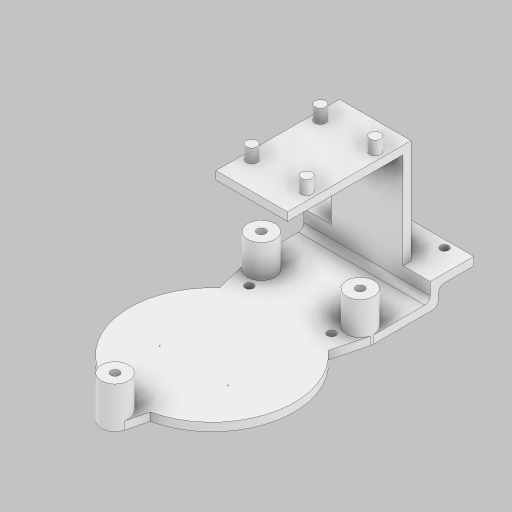
# Autodesk Inventor part: BASE_LIDAR_V4
Saved by Autodesk Inventor 2024.2 (Build 282272000, 272)
## iProperties
Created: 2024-07-17
Part Number: BASE_LIDAR_V4
Material: ABS Plastic
Document SubType Name: Modeling
Designer: jrcer
Density: 1.06 g/cm^3
Appearance: Smooth - White
Mass: 26.2686 g
Surface Area: 178.873 cm^2
Volume: 24.7817 cm^3
Author: jrcer
Autodesk Inventor part; units mm, degrees
ref_plane "YZ Plane" through (0, 0, 0) normal (1, 0, 0) x (0, 1, 0)
ref_plane "XZ Plane" through (0, 0, 0) normal (0, 1, 0) x (-1, 0, 0)
ref_plane "XY Plane" through (0, 0, 0) normal (0, 0, 1) x (1, 0, 0)
sketch "Sketch1" plane through (0, 0, 0) normal (0, 1, 0) x (-1, 0, 0)
  circle A0 centre (0, 35.3) radius 1.55
  circle A1 centre (18, -36) radius 1.55
  circle A2 centre (-18, -36) radius 1.55
  circle A3 centre (0, 35.3) radius 5
  circle A4 centre (18, -36) radius 5
  circle A5 centre (-18, -36) radius 5
  point P0 (0, 0)
  dimension "d0" = 35.3
  dimension "d1" = 36
  dimension "d2" = 3.1
  dimension "d3" = 10
  dimension "d4" = 36
  dimension "d5" = 18
  constraints: 6 centre point, 4 equal radius, 3 coincident, 1 horizontal alignment, 1 vertical alignment
  measures "d0" distance of A0.centre point (0, 0)
  measures "d1" vertical distance of A2.centre point (0, 0)
  measures "d2" diameter of A0
  measures "d3" diameter of A3
  measures "d4" distance of A2.centre A1.centre
  measures "d5" horizontal distance of point (0, 0) A2.centre
extrude "Extrusion1" add sketch "Sketch1" along normal blind 12
sketch "Sketch2" plane through (0, 0, 35.3) normal (0, -1, 0) x (1, 0, 0)
  circle A0 centre (0, 0) radius 5 projected
  circle A1 centre (0, 0) radius 1.55 projected
  circle A2 centre (-18, -71.3) radius 1.55 projected
  circle A3 centre (-18, -71.3) radius 5 projected
  circle A4 centre (18, -71.3) radius 1.55 projected
  circle A5 centre (18, -71.3) radius 5 projected
  line L0 (-22.8479, -70.0761) -> (-4.8479, 1.2239)
  line L1 (22.8479, -70.0761) -> (4.8479, 1.2239)
  line L2 (-18, -76.3) -> (18, -76.3)
  circle A6 centre (0, -35.3) radius 2.1
  circle A7 centre (0, -35.3) radius 30
  circle A8 centre (0, -22.8) radius 1.5
  circle A9 centre (-7.5, -22.8) radius 1.5
  circle A10 centre (-15, -22.8) radius 1.5
  circle A11 centre (7.5, -22.8) radius 1.5
  circle A12 centre (15, -22.8) radius 1.5
  circle A13 centre (-15, -63.9) radius 1.5
  circle A14 centre (15, -63.9) radius 1.5
  line L3 (-12.5, -46.4) -> (12.5, -46.4)
  line L4 (12.5, -46.4) -> (12.5, -26.4)
  line L5 (12.5, -26.4) -> (-12.5, -26.4)
  line L6 (-12.5, -26.4) -> (-12.5, -46.4)
  line L7 (-12.5, -46.4) -> (12.5, -26.4) construction
  line L8 (12.5, -46.4) -> (-12.5, -26.4) construction
  circle A15 centre (-12.5, -26.4) radius 2.05
  circle A16 centre (12.5, -46.4) radius 2.05
  circle A17 centre (12.5, -26.4) radius 2.05
  circle A18 centre (-12.5, -46.4) radius 2.05
  line L9 (-23, -71.3) -> (-23, -94.8)
  line L10 (-23, -94.8) -> (23, -94.8)
  line L11 (23, -94.8) -> (23, -71.3)
  circle A19 centre (18, -71.3) radius 5 projected
  circle A20 centre (-18, -71.3) radius 5 projected
  point P0 (6.6853, -6.0544)
  point P1 (19.7659, -57.8679)
  point P2 (-6.6853, -6.0544)
  point P3 (-19.7659, -57.8679)
  point P4 (0, -36.4)
  point P5 (12.5, -29.0869)
  point P6 (12.3376, -28.4436)
  point P7 (12.5, -28.45)
  point P8 (-12.5, -29.0869)
  point P9 (-12.5, -28.45)
  point P10 (-12.3376, -28.4436)
  dimension "d8" = 4.2
  dimension "d78" = 60
  dimension "d79" = 12.5
  dimension "d80" = 7.5
  dimension "d81" = 7.5
  dimension "d82" = 3
  dimension "d83" = 7.5
  dimension "d84" = 7.5
  dimension "d85" = 41.1
  dimension "d86" = 27.5
  dimension "d87" = 25
  dimension "d88" = 20
  dimension "d89" = 4.1
  dimension "d91" = 18.5
  constraints: 24 end point, 13 centre point, 9 equal radius, 8 point on circle, 7 tangent, 6 coincident, 5 horizontal alignment, 4 vertical alignment, 3 perpendicular, 2 horizontal, 2 midpoint, 2 parallel, 1 point on line, 1 vertical
  measures "d8" diameter of A6
  measures "d78" diameter of A7
  measures "d79" distance of A8.centre point (0, -35.3)
  measures "d80" distance of A8.centre A9.centre
  measures "d81" distance of A10.centre A9.centre
  measures "d82" diameter of A8
  measures "d83" distance of A11.centre A8.centre
  measures "d84" distance of A11.centre A12.centre
  measures "d85" distance of A10.centre A13.centre
  measures "d86" vertical distance of point (0, -36.4) A13.centre
  measures "d87" distance of L3.start L3.end
  measures "d88" distance between parallel lines of L5 L3
  measures "d89" diameter of A15
  measures "d91" distance between parallel lines of L2 L10
extrude "Extrusion2" add sketch "Sketch2" along normal blind 3 contours A0 | A0 L1 A7 L0 | A7 L1 L4 A17 | L1 A17 L5 A15 L0 A7 | L0 A15 L6 A7 | A17 L4 L5 L1 | L1 L5 A17 | A15 L5 L0 | L0 L5 L6 A15 | A7 L1 A5 L2 A3 L0 | L0 L6 A18 L3 A16 L4 L1 A7 | L5 L4 A17 L1 | L1 A17 L5 | A17 L1 L4 A16 L3 A18 L6 L0 A15 L5 | L5 A15 L0 | L0 A15 L6 L5 | A3 | A5 | A3 L2 A5 L11 L10 L9 | A18 L3 L6 | L6 L3 A18 | A16 L3 L4 | L4 L3 A16 | A6 | A8 | A9 | A10 | A11 | A12
sketch "Sketch6" plane through (0, 0, 35.3) normal (0, 1, 0) x (1, 0, 0)
  line L0 (-23, 71.3) -> (-23, 94.8) construction
  line L1 (23, 94.8) -> (23, 71.3) construction
  line L2 (-23, 94.8) -> (23, 94.8) construction
  circle A0 centre (-18, 71.3) radius 5 construction
  circle A1 centre (18, 71.3) radius 5 construction
  line L3 (-23, 94.8) -> (23, 94.8)
  line L4 (23, 94.8) -> (23, 91.8)
  line L5 (23, 91.8) -> (-23, 91.8)
  line L6 (-23, 91.8) -> (-23, 94.8)
  arc A2 (23, 71.3) -> (22.8479, 70.0761) centre (18, 71.3) ccw construction
  arc A3 (-22.8479, 70.0761) -> (-23, 71.3) centre (-18, 71.3) ccw construction
  point P0 (0, 35.3)
  point P1 (13.0382, 71.9166)
  point P2 (-13.0382, 71.9166)
  dimension "d94" = 3
  constraints: 8 end point, 3 point on line, 2 parallel, 2 point on circle, 1 horizontal, 1 perpendicular
  measures "d94" distance of L5.end L3.start
extrude "Extrusion6" add sketch "Sketch6" along normal blind 3.42
sketch "Sketch7" plane through (0, 3.42, 35.3) normal (0, 1, 0) x (1, 0, 0)
  line L0 (-23, 107.7) -> (23, 107.7)
  line L1 (23, 107.7) -> (23, 91.8)
  line L2 (23, 91.8) -> (-23, 91.8)
  line L3 (-23, 91.8) -> (-23, 107.7)
  line L4 (-23, 91.8) -> (23, 91.8) projected
  line L5 (-23, 71.3) -> (-23, 91.8) projected
  point P0 (0, 35.3)
  point P1 (0, 91.8)
  point P2 (0, 91.8)
  point P3 (-23, 94.8)
  dimension "d106" = 15.9
  constraints: 8 end point, 2 collinear, 2 midpoint, 2 parallel, 1 coincident, 1 horizontal, 1 perpendicular
  measures "d106" distance of L0.end L1.end
extrude "Extrusion8" add sketch "Sketch7" along normal blind 3
sketch "Sketch8" plane through (0, 6.42, 35.3) normal (0, 1, 0) x (1, 0, 0)
  circle A0 centre (-15, 105) radius 1.5
  circle A1 centre (15, 105) radius 1.5
  circle A2 centre (-15, 63.9) radius 1.5 construction
  circle A3 centre (15, 63.9) radius 1.5 construction
  line L0 (23, 107.7) -> (-23, 107.7) construction
  point P0 (0, 35.3)
  dimension "d107" = 2.7
  dimension "d108" = 3
  dimension "d109" = 3
  constraints: 2 centre point, 2 vertical alignment, 1 horizontal alignment
  measures "d107" distance from line of L0 A0.centre
  measures "d108" diameter of A0
  measures "d109" diameter of A1
extrude "Extrusion9" cut sketch "Sketch8" against normal blind 3
fillet "Fillet3" radius 2 3 edges at (0, 0, -56.5) (0, 3.42, -59.5) (0, -3, -59.5)
sketch "Sketch9" plane through (0, 6.42, 35.3) normal (0, 1, 0) x (1, 0, 0)
  line L0 (-23, 107.7) -> (-23, 91.8) construction
  line L1 (23, 91.8) -> (23, 107.7) construction
  circle A0 centre (-18, 71.3) radius 5 construction
  circle A1 centre (18, 71.3) radius 5 construction
  line L2 (-23, 91.8) -> (23, 91.8) projected
  line L3 (-13.0382, 91.8) -> (13.0382, 91.8)
  line L4 (13.0382, 91.8) -> (13.0382, 94.8)
  line L5 (13.0382, 94.8) -> (-13.0382, 94.8)
  line L6 (-13.0382, 94.8) -> (-13.0382, 91.8)
  arc A2 (-22.8479, 70.0761) -> (-23, 71.3) centre (-18, 71.3) ccw projected
  arc A3 (23, 71.3) -> (22.8479, 70.0761) centre (18, 71.3) ccw projected
  point P0 (0, 35.3)
  point P1 (-13.0382, 71.9166)
  point P2 (13.0382, 71.9166)
  point P3 (13.0382, 91.8)
  dimension "d115" = 3
  constraints: 8 end point, 2 parallel, 2 point on circle, 2 vertical alignment, 1 horizontal, 1 perpendicular, 1 point on line
  measures "d115" distance of L4.end L3.end
extrude "Extrusion10" add sketch "Sketch9" along normal blind 35
sketch "Sketch10" plane through (13.0382, 6.42, -59.5) normal (0, 0, -1) x (-1, 0, 0)
  line L0 (26.0763, 0) -> (0, 0) construction
  line L1 (26.0763, 0) -> (26.0763, 35) construction
  line L2 (0, 35) -> (26.0763, 35) construction
  line L3 (0, 0) -> (0, 35) construction
  line L4 (0, 35) -> (26.0763, 35)
  line L5 (26.0763, 35) -> (26.0763, 38)
  line L6 (26.0763, 38) -> (0, 38)
  line L7 (0, 38) -> (0, 35)
  point P0 (13.0382, -6.42)
  dimension "d118" = 3
  constraints: 8 end point, 2 parallel, 1 collinear, 1 horizontal, 1 perpendicular
  measures "d118" distance between parallel lines of L4 L6
extrude "Extrusion11" add sketch "Sketch10" against normal blind 45
sketch "Sketch11" plane through (-13.0382, 44.42, -59.5) normal (0, 1, 0) x (1, 0, 0)
  line L0 (0, 0) -> (26.0763, 0) projected
  line L1 (0, 0) -> (0, -45) projected
  line L2 (26.0763, -45) -> (0, -45) projected
  line L3 (26.0763, 0) -> (26.0763, -45) projected
  line L4 (3.0382, -35) -> (23.0382, -35)
  line L5 (23.0382, -35) -> (23.0382, -10)
  line L6 (23.0382, -10) -> (3.0382, -10)
  line L7 (3.0382, -10) -> (3.0382, -35)
  line L8 (3.0382, -35) -> (23.0382, -10) construction
  line L9 (23.0382, -35) -> (3.0382, -10) construction
  circle A0 centre (3.0382, -35) radius 2
  circle A1 centre (3.0382, -10) radius 2
  circle A2 centre (23.0382, -10) radius 2
  circle A3 centre (23.0382, -35) radius 2
  point P0 (13.0382, -59.5)
  point P1 (13.0382, -22.5)
  point P2 (3.0382, -22.5)
  point P3 (26.0763, -22.5)
  point P4 (13.0382, -35)
  point P5 (13.0382, -45)
  dimension "d121" = 20
  dimension "d122" = 25
  dimension "d123" = 4
  constraints: 12 end point, 6 midpoint, 4 centre point, 4 coincident, 3 equal radius, 2 parallel, 1 horizontal, 1 horizontal alignment, 1 perpendicular, 1 vertical alignment
  measures "d121" distance of L6.end L5.end
  measures "d122" distance of L6.end L4.start
  measures "d123" diameter of A0
extrude "Extrusion12" add sketch "Sketch11" along normal blind 5 contours L7 A0 L4 | L4 A0 L7 | A3 L5 L4 | L4 L5 A3 | A1 L6 L7 | L7 L6 A1 | A2 L6 L5 | L5 L6 A2
equation "\"d5\" = 0.5 * d4"
body "Solid1"
